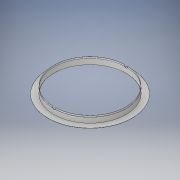
# Autodesk Inventor part: Layer2_Bottom
Saved by Autodesk Inventor 2017 (Build 210142000, 142)
## iProperties
Created: 2016-12-23
Part Number: Layer2_Bottom
Material: Generic
Document SubType Name: Modeling
Designer: David Kopala
Density: 1 g/cm^3
Appearance: Default
Author: David Kopala
Autodesk Inventor part; units mm, degrees
ref_plane "YZ Plane" through (0, 0, 0) normal (1, 0, 0) x (0, 1, 0)
ref_plane "XZ Plane" through (0, 0, 0) normal (0, 1, 0) x (-1, 0, 0)
sketch "Sketch1" plane through (0, 0, 0) normal (1, 0, 0) x (0, 1, 0)
  line L0 (0, 0) -> (1.9826, 0)
  line L1 (0, 149.225) -> (25.4, 149.225)
  line L2 (0, 149.225) -> (0, 174.625)
  line L3 (0, 174.625) -> (0.7937, 174.625)
  line L4 (0.7937, 174.625) -> (0.7937, 150.0187)
  line L5 (0.7937, 150.0187) -> (22.225, 150.0187)
  line L6 (25.4, 149.6219) -> (25.4, 149.225)
  line L7 (25.4, 149.225) -> (28.575, 149.225)
  line L8 (28.575, 149.225) -> (28.575, 149.6219)
  line L9 (28.575, 149.6219) -> (22.225, 149.6219)
  line L10 (22.225, 149.6219) -> (22.225, 150.0187)
  point P0 (0.3969, 174.625)
  dimension "d0" = 25.4
  dimension "d1" = 149.225
  dimension "d2" = 25.4
  dimension "d3" = 0.7937
  dimension "d4" = 24.6062
  dimension "d5" = 3.175
  dimension "d6" = 6.35
  constraints: 22 end point, 7 perpendicular, 2 horizontal, 2 midpoint, 2 vertical
  measures "d0" distance of L1.start L1.end
  measures "d1" distance between parallel lines of L0 L1
  measures "d2" distance of L1.start L2.end
  measures "d3" distance of L2.end L3.end
  measures "d4" distance of L3.end L4.end
  measures "d5" distance of L1.end L7.end
  measures "d6" distance of L8.end L9.end
revolve "Revolution1" add sketch "Sketch1" angle 360 about axis through (0, 0, 0) along (0, 1, 0)
ref_plane "Work Plane1" through (0, 0.3969, 174.625) normal (0, 0, 1) x (1, 0, 0)
sketch "Sketch2" plane through (0, 0.3969, 174.625) normal (0, 0, 1) x (1, 0, 0)
  line L0 (149.6219, 28.1781) -> (-149.6219, 28.1781) projected
  arc A0 (-6.35, 25.0031) -> (6.35, 25.0031) centre (0, 25.0031) ccw
  line L1 (-6.35, 25.0031) -> (-6.35, 28.1781)
  line L2 (6.35, 25.0031) -> (6.35, 28.1781)
  line L3 (149.225, 28.1781) -> (-149.225, 28.1781) projected
  line L4 (-6.35, 28.1781) -> (6.35, 28.1781)
  point P0 (0, -0.3969)
  dimension "d8" = 3.175
  dimension "d9" = 0
  dimension "d10" = 12.7
  constraints: 6 end point, 2 point on circle, 2 point on line, 1 centre point, 1 coincident, 1 collinear, 1 perpendicular, 1 tangent, 1 vertical
  measures "d8" distance from line of L0 point (0, 25.003)
  measures "d9" horizontal distance of point (0, -0.397) point (0, 25.003)
  measures "d10" diameter of A0
extrude "Extrusion1" cut sketch "Sketch2" against normal through all
body "Solid1"
